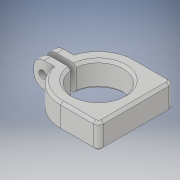
# Autodesk Inventor part: BasicMount 19.5mm
Saved by Autodesk Inventor 2019.3 (Build 233278000, 278)
## iProperties
Created: 2019-04-04
Part Number: BasicMount 19.5mm
Material: Типовые
Document SubType Name: Modeling
Designer: Andrew
Density: 1 g/cm^3
Appearance: По умолчанию
Author: Andrew
Autodesk Inventor part; units mm, degrees
ref_plane "YZ Plane" through (0, 0, 0) normal (1, 0, 0) x (0, 1, 0)
ref_plane "XZ Plane" through (0, 0, 0) normal (0, 1, 0) x (-1, 0, 0)
ref_plane "XY Plane" through (0, 0, 0) normal (0, 0, 1) x (1, 0, 0)
sketch "Эскиз1" plane through (0, 0, 0) normal (0, 1, 0) x (-1, 0, 0)
  arc A0 (9.8249, 1.217) -> (9.8505, -0.9889) centre (0, 0) ccw
  line L0 (-15.0002, 15) -> (-15.0002, -15)
  line L1 (-15.0002, 15) -> (0, 15)
  line L2 (-15.0002, -15) -> (0, -15)
  line L3 (9.8249, 1.217) -> (16.2051, 1.217)
  line L4 (13.6718, -0.9889) -> (9.8505, -0.9889)
  arc A1 (0, -15) -> (14.5136, -3.7889) centre (0, 0) ccw
  arc A2 (14.4521, 4.017) -> (0, 15) centre (0, 0) ccw
  line L5 (9.8505, -0.9889) -> (21.6521, -0.9889)
  line L6 (21.6521, -0.9889) -> (21.6521, -3.7889)
  line L7 (21.6521, -3.7889) -> (14.5136, -3.7889)
  line L8 (9.8249, 1.217) -> (21.6265, 1.217)
  line L9 (21.6265, 1.217) -> (21.6265, 4.017)
  line L10 (21.6265, 4.017) -> (14.4521, 4.017)
  point P0 (15, 0)
  dimension "d0" = 19.8
  dimension "d2" = 30
  dimension "d5" = 2.8
  dimension "d6" = 2.8
  constraints: 22 end point, 6 point on circle, 5 parallel, 4 horizontal, 3 centre point, 2 coincident, 2 perpendicular, 2 tangent, 1 concentric, 1 vertical
  measures "d0" diameter of A0
  measures "d2" distance of L0.start L0.end
  measures "d5" distance between parallel lines of L7 L5
  measures "d6" distance of L8.end L9.end
extrude "Выдавливание1" add sketch "Эскиз1" along normal blind 10
fillet "Сопряжение1" radius 4 4 edges at (-21.6265, 10, 2.617) (-21.6521, 10, -2.3889) (-21.6265, 0, 2.617) (-21.6521, 0, -2.3889)
sketch "Эскиз3" plane through (-14.4521, 0, 4.017) normal (0, 0, 1) x (1, 0, 0)
  arc A0 (-7.1744, 4) -> (-3.1744, 0) centre (-3.1744, 4) ccw projected
  line L0 (-3.1744, 0) -> (0, 0) projected
  line L1 (0, 0) -> (0, 10) projected
  line L2 (-3.1744, 10) -> (0, 10) projected
  arc A1 (-3.1744, 10) -> (-7.1744, 6) centre (-3.1744, 6) ccw projected
  line L3 (-7.1744, 4) -> (-7.1744, 6) projected
  line L4 (-7.1744, 5) -> (-3.6744, 5) construction
  point P0 (14.4521, 0)
  dimension "d20" = 3.5
  constraints: 2 end point, 1 coincident, 1 horizontal, 1 midpoint
  measures "d20" distance of L4.start L4.end
hole "Отверстие2" at (-18.1265, 5, 4.017) direction (0, 0, -1) diameter 3 depth 8 tip angle 118
fillet "Сопряжение2" radius 2 2 edges at (15.0002, 5, 15) (15.0002, 5, -15)
chamfer "Фаска1" distance 1 angle 45 16 edges at (9.8993, 10, -0.1148) (9.8993, 0, -0.1148) (6.5001, 10, 15) (14.4144, 10, 14.4142) (15.0002, 10, 0) (14.4144, 10, -14.4142) (6.5001, 10, -15) (-9.1697, 10, -11.8708) (-9.0759, 10, 11.9427) (6.5001, 0, 15) (14.4144, 0, 14.4142) (15.0002, 0, 0) (14.4144, 0, -14.4142) (6.5001, 0, -15) (-9.1697, 0, -11.8708) (-9.0759, 0, 11.9427)
